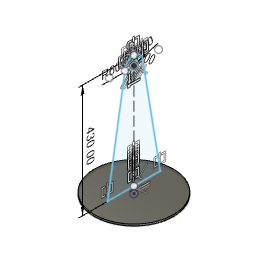
cannon_base (Autodesk Fusion 360 design; units mm, degrees)
Autodesk Fusion 360 part; units mm, degrees
sketch "Sketch1" plane through (0, 0, 0) normal (0, 0, 1) x (1, 0, 0)
  circle A0 centre (0, 0) radius 150
  dimension "d1" = 300
  constraint coincident A0.centre origin
  measures "d1" diameter of A0
extrude "Extrude1" add sketch "Sketch1" along normal blind 6.2
sketch "Sketch3" plane through (0, 0, 0) normal (1, 0, 0) x (0, 1, 0)
  line L0 (0, 25) -> (100, 25)
  line L1 (0, 25) -> (0, 455) construction
  circle A0 centre (0, 421) radius 14
  line L2 (0, 0) -> (0, 25) construction
  line L3 (0, 421) -> (-14, 421) construction
  line L4 (0, 421) -> (14, 421) construction
  line L5 (14, 421) -> (34, 421) construction
  line L6 (34.6123, 417.326) -> (100, 25)
  arc A1 (33.9262, 423.2389) -> (0, 455) centre (0, 421) ccw
  line L7 (-14, 421) -> (-34, 421) construction
  arc A2 (33.9262, 423.2389) -> (34.6123, 417.326) centre (93.796, 427.1899) ccw
  arc A3 (0, 455) -> (-33.9262, 423.2389) centre (0, 421) ccw
  line L8 (-34.6123, 417.326) -> (-100, 25)
  line L9 (0, 25) -> (-100, 25)
  arc A4 (-34.6123, 417.326) -> (-33.9262, 423.2389) centre (-93.796, 427.1899) ccw
  dimension "d11" = 430
  dimension "d13" = 28
  dimension "d14" = 20
  dimension "d15" = 60
  constraint horizontal L0
  constraint perpendicular L0 L1
  constraint concentric A0 A1
  constraint coincident L2.start origin
  constraint perpendicular L0 L2
  constraint coincident A0.centre L3.start
  constraint coincident A0 L3.end
  constraint perpendicular L1 L3
  constraint coincident A0 L4.end
  constraint perpendicular L1 L4
  constraint parallel L4 L5
  constraint parallel L3 L7
  constraint coincident L5.end L6
  constraint coincident L5.end A1
  constraint tangent L6 A2
  constraint tangent A1 A2
  constraint symmetric L0.start L1 L2.end
  constraint symmetric L0.end L1 L8.end
  constraint symmetric A1.end L1 A3.start
  constraint symmetric L1 A1 A3
  constraint symmetric L1 L6.start L8.start
  constraint symmetric L1 A1.start A3.end
  constraint symmetric L1 A2 A4
  measures "d11" distance of L0.start L1.end
  measures "d13" diameter of A0
  measures "d14" distance of A0 A1
  measures "d15" radius of A2
